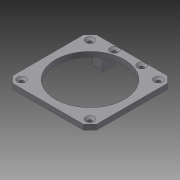
# Autodesk Inventor part: Крышка
Saved by Autodesk Inventor 2022 (Build 260153000, 153)
## iProperties
RuleStatus: InUse
Part Number: Крышка
Checked By: Якушев
Engr Approved By: Малов
Material: По умолчанию1
Document SubType Name: Modeling
Mfg Approved By: Судаков
Designer: Смирнов
Density: 1 g/cm^3
Appearance: По умолчанию1
AfterMaterialChange0: Материал
BeforeDocSave0: Материал
AfterAnyiPropertyChange0: Материал
Материал: По умолчанию1
Author: Смирнов
Autodesk Inventor part; units mm, degrees
ref_plane "YZ Plane" through (0, 0, 0) normal (1, 0, 0) x (0, 1, 0)
ref_plane "XZ Plane" through (0, 0, 0) normal (0, 1, 0) x (-1, 0, 0)
ref_plane "РабПлоскость1" through (0, 0, 75.2) normal (0, 0, 1) x (1, 0, 0)
sketch "Эскиз1" plane through (0, 0, 75.2) normal (0, 0, 1) x (1, 0, 0)
  circle A0 centre (26.4645, -26.4645) radius 1.95 construction
  circle A1 centre (-26.4645, 26.4645) radius 1.95 construction
  circle A2 centre (26.4645, 26.4645) radius 1.95 construction
  circle A3 centre (-26.4645, -26.4645) radius 1.95 construction
  circle A4 centre (15.35, -15.35) radius 1.7 construction
  circle A5 centre (-15.35, 15.35) radius 1.7 construction
  circle A6 centre (15.35, 15.35) radius 1.7 construction
  circle A7 centre (-15.35, -15.35) radius 1.7 construction
  line L0 (-32.5, 27.5) -> (-32.5, -27.5) projected
  line L1 (-27.5, 32.5) -> (-32.5, 27.5) projected
  line L2 (27.5, 32.5) -> (-27.5, 32.5) projected
  line L3 (32.5, 27.5) -> (27.5, 32.5) projected
  line L4 (32.5, -27.5) -> (32.5, 27.5) projected
  line L5 (27.5, -32.5) -> (32.5, -27.5) projected
  line L6 (-27.5, -32.5) -> (27.5, -32.5) projected
  line L7 (-32.5, -27.5) -> (-27.5, -32.5) projected
  circle A8 centre (0, 0) radius 11.5 construction
  circle A9 centre (0, 0) radius 26.7 projected
  point P0 (0, 0)
extrude "Выдавливание1" add sketch "Эскиз1" along normal blind 4
sketch "Эскиз2" plane through (0, 0, 79.2) normal (0, 0, 1) x (1, 0, 0)
  circle A0 centre (26.4645, 26.4645) radius 2.25 projected
  circle A1 centre (26.4645, -26.4645) radius 2.25 projected
  circle A2 centre (-26.4645, -26.4645) radius 2.25 projected
  circle A3 centre (-26.4645, 26.4645) radius 1.95 projected
  circle A4 centre (10.5, 29.5) radius 2.25 construction
  circle A5 centre (-10.5, 29.5) radius 1.65 construction
  constraints: 2 centre point, 2 coincident, 4 other
hole "Отверстие1" at (26.4645, 26.4645, 79.2) at (-26.4645, 26.4645, 79.2) at (26.4645, -26.4645, 79.2) at (-26.4645, -26.4645, 79.2) at (10.5, 29.5, 79.2) at (-10.5, 29.5, 79.2) direction (0, 0, -1) diameter 3.4 end through all countersink diameter 6 countersink angle 90 clearance for "с потайной головкой ГОСТ 12876-67" size "M3" standard "ГОСТ"
sketch "Эскиз3" plane through (0, 0, 75.2) normal (0, 0, -1) x (-1, 0, 0)
  line L0 (-21.5, 32.5) -> (-13.5, 32.5) construction
  line L1 (-13.5, 32.5) -> (-13.5, 22.5) construction
  line L2 (-13.5, 22.5) -> (-21.5, 22.5) construction
  line L3 (-21.5, 22.5) -> (-21.5, 32.5) construction
  line L4 (13.5, 32.5) -> (21.5, 32.5) construction
  line L5 (21.5, 32.5) -> (21.5, 22.5) construction
  line L6 (21.5, 22.5) -> (13.5, 22.5) construction
  line L7 (13.5, 22.5) -> (13.5, 32.5) construction
  line L8 (0, 0) -> (0, 42.6658) construction
  line L9 (-27.5, 32.5) -> (27.5, 32.5) construction
  line L10 (-21.3, 32.5) -> (-13.7, 32.5)
  line L11 (-13.7, 32.5) -> (-13.7, 23.5)
  line L12 (-13.7, 23.5) -> (-21.3, 23.5)
  line L13 (-21.3, 23.5) -> (-21.3, 32.5)
  line L14 (13.7, 32.5) -> (21.3, 32.5)
  line L15 (21.3, 32.5) -> (21.3, 23.5)
  line L16 (21.3, 23.5) -> (13.7, 23.5)
  line L17 (13.7, 23.5) -> (13.7, 32.5)
  dimension "d9" = 10
  dimension "d10" = 0.2
  dimension "d11" = 0.2
  dimension "d12" = 9
  constraints: 34 end point, 8 parallel, 5 point on line, 4 horizontal, 4 perpendicular, 1 vertical, 8 other
  measures "d9" distance of L4.end L5.end
  measures "d10" distance between parallel lines of L7 L17
  measures "d11" distance between parallel lines of L15 L5
  measures "d12" distance of L16.end L14.start
extrude "Выдавливание2" add sketch "Эскиз3" along normal blind 12
sketch "Эскиз4" plane through (-27.5, 32.5, 79.2) normal (0, 1, 0) x (1, 0, 0)
  arc A0 (14, 16) -> (6, 16) centre (10, 16) ccw
  arc A1 (49, 16) -> (41, 16) centre (45, 16) ccw
  circle A2 centre (45, 16) radius 4
  circle A3 centre (10, 16) radius 4
  point P0 (27.5, 79.2)
  constraints: 4 point on circle, 2 centre point, 2 coincident, 14 other
extrude "Выдавливание3" cut sketch "Эскиз4" against normal through all
fillet "Сопряжение1" radius 0.2 4 edges at (-21.3, 28, 64.449) (-13.7, 28, 64.449) (13.7, 28, 64.449) (21.3, 28, 64.449)
sketch "Эскиз5" plane through (0, 0, 75.2) normal (0, 0, -1) x (-1, 0, 0)
  line L0 (14.0714, 23.5) -> (14.0714, 32.5) construction
  line L1 (20.9286, 23.5) -> (14.0714, 23.5) construction
  line L2 (20.9286, 32.5) -> (20.9286, 23.5) construction
  line L3 (14.0714, 32.5) -> (20.9286, 32.5) construction
  line L4 (-20.9286, 23.5) -> (-20.9286, 32.5) construction
  line L5 (-14.0714, 23.5) -> (-20.9286, 23.5) construction
  line L6 (-14.0714, 32.5) -> (-14.0714, 23.5) construction
  line L7 (-20.9286, 32.5) -> (-14.0714, 32.5) construction
  line L8 (20.9286, 23.5) -> (14.0714, 32.5) construction
  line L9 (19, 32.5) -> (16, 32.5)
  line L10 (16, 32.5) -> (16, 23.5)
  line L11 (16, 23.5) -> (19, 23.5)
  line L12 (19, 23.5) -> (19, 32.5)
  line L13 (19, 32.5) -> (16, 23.5) construction
  line L14 (16, 32.5) -> (19, 23.5) construction
  point P0 (0, 0)
  point P1 (17.5, 28)
  dimension "d18" = 3
  constraints: 14 end point, 3 midpoint, 3 parallel, 1 horizontal, 1 perpendicular
  measures "d18" distance between parallel lines of L12 L10
extrude "Выдавливание4" add sketch "Эскиз5" along normal blind 9
mirror "Зеркальное отражение1" about plane through (0, 0, 0) normal (1, 0, 0) of "Выдавливание4"
equation "\"d11\" = d10"
